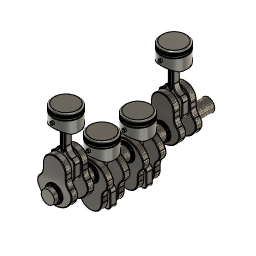
piston v3 (Autodesk Fusion 360 design; units mm, degrees)
Autodesk Fusion 360 part; units mm, degrees
note: some values were not read from the file. Set by a fixed rule: which face or edge a step refers to.
sketch "Sketch1" plane through (0, 0, 0) normal (0, 1, 0) x (1, 0, 0) in component "piston"
  line L0 (0, 0) -> (40, 0)
  line L1 (40, 0) -> (40, -55)
  line L2 (40, -55) -> (0, -55)
  line L3 (0, -55) -> (0, 0)
  line L4 (40, -48) -> (36, -48)
  line L5 (36, -48) -> (36, -46)
  line L6 (36, -46) -> (40, -46)
  line L7 (40, -46) -> (40, -48)
  line L8 (40, -44) -> (36, -44)
  line L9 (36, -44) -> (36, -42)
  line L10 (36, -42) -> (40, -42)
  line L11 (40, -42) -> (40, -44)
  line L12 (40, -38) -> (36, -38)
  line L13 (36, -38) -> (36, -36)
  line L14 (36, -36) -> (40, -36)
  line L15 (40, -36) -> (40, -38)
  dimension "d1" = 55
  dimension "d2" = 40
  dimension "d3" = 7
  dimension "d4" = 2
  dimension "d5" = 4
  dimension "d6" = 2
  dimension "d7" = 2
  dimension "d8" = 2
  dimension "d9" = 4
  dimension "d10" = 4
  dimension "d11" = 4
  constraint horizontal L0
  constraint vertical L1
  constraint horizontal L2
  constraint vertical L3
  constraint coincident L0.start L3.end
  constraint horizontal L4
  constraint vertical L5
  constraint horizontal L6
  constraint vertical L7
  constraint coincident L1 L4.start
  constraint horizontal L8
  constraint vertical L9
  constraint horizontal L10
  constraint vertical L11
  constraint coincident L1 L8.start
  constraint horizontal L12
  constraint vertical L13
  constraint horizontal L14
  constraint vertical L15
  constraint coincident L1 L12.start
  measures "d1" distance of L0.start L2.end
  measures "d2" distance of L0.start L0.end
  measures "d3" distance of L2 L4
  measures "d4" distance of L6 L8
  measures "d5" distance of L10 L12
  measures "d6" distance of L4.end L5.end
  measures "d7" distance of L8.end L9.end
  measures "d8" distance of L12.end L13.end
  measures "d9" distance of L4.start L4.end
  measures "d10" distance of L8.start L8.end
  measures "d11" distance of L12.start L12.end
revolve "Revolve1" add sketch "Sketch1" angle 360 about axis through (0, 0, 55) along (0, 0, -1) contours L0 L1 L2 L3 L4 L5 L6 L8 L9 L10 L12 L13 L14 makes body 1 in component "piston"
fillet "Fillet1" radius 5 1 edges at (-37.2931, -14.4646, 55) on bodies 1 in component "piston"
sketch "Sketch2" plane through (0, 0, 0) normal (0, 0, 1) x (1, 0, 0) in component "piston"
  circle A0 centre (0, 0) radius 35
  dimension "d15" = 70
  constraint coincident A0.centre origin
  measures "d15" diameter of A0
extrude "Extrude1" cut sketch "Sketch2" along normal blind 50 bodies 1 in component "piston"
sketch "Sketch3" plane through (0, 0, 0) normal (0, 1, 0) x (1, 0, 0) in component "piston"
  line L0 (-40, 0) -> (40, 0)
  line L1 (-40, -36) -> (40, -36)
  line L2 (0, 0) -> (0, -10)
  arc A0 (-35.5, 0) -> (35.5, 0) centre (0, 58.0125) ccw
  circle A1 centre (0, -24) radius 5
  dimension "d18" = 4.5
  dimension "d19" = 4.5
  dimension "d20" = 10
  dimension "d21" = 24
  dimension "d22" = 10
  constraint coincident L2.start origin
  constraint perpendicular L0 L2
  constraint coincident L2.end A0
  constraint coincident L0 A0.end
  constraint coincident L0 A0.start
  measures "d18" distance of L0.start A0.start
  measures "d19" distance of L0.end A0.end
  measures "d20" diameter of A1
  measures "d21" distance of L2.start A1.centre
  measures "d22" distance of L2.start L2.end
extrude "Extrude2" cut sketch "Sketch3" along normal mid plane 90 bodies 1 in component "piston"
pattern_linear "R-Pattern1" count 4 spacing 250 along (0, -1, 0) of bodies 1 makes body 2 at (-8.1193, -284.0452, 27.7018) makes body 3 at (-8.1193, -534.0452, 27.7018) makes body 4 at (-8.1193, -784.0452, 27.7018) in component "piston"
sketch "Sketch1 (2)" plane through (0, 0, 0) normal (0, 1, 0) x (1, 0, 0) in component "connecting rod"
  circle A0 centre (0, -50) radius 8.5
  circle A1 centre (0, -50) radius 5
  circle A2 centre (0, 75) radius 22.5
  line L0 (8.5, -50) -> (8.5, 25)
  line L1 (0, 75) -> (36, 75)
  line L2 (36, 75) -> (36, 50)
  line L3 (36, 50) -> (33.5, 50)
  arc A3 (33.5, 50) -> (8.5, 25) centre (33.5, 25) ccw
  line L4 (0, 75) -> (0, 20) construction
  line L5 (-8.5, -50) -> (-8.5, 25)
  arc A4 (-8.5, 25) -> (-33.5, 50) centre (-33.5, 25) ccw
  line L6 (-36, 75) -> (-36, 50)
  line L7 (-36, 50) -> (-33.5, 50)
  line L8 (0, 75) -> (-36, 75)
  line L9 (-36, 75) -> (36, 75)
  line L10 (36, 75) -> (36, 107.5)
  line L11 (36, 107.5) -> (-36, 107.5)
  line L12 (-36, 107.5) -> (-36, 75)
  circle A5 centre (0, -35) radius 4.75
  circle A6 centre (0, 37.5) radius 4.75
  line L13 (-4.75, -35) -> (-4.75, 37.5)
  line L14 (4.75, 37.5) -> (4.75, -35)
  dimension "d29" = 10
  dimension "d30" = 17
  dimension "d31" = 45
  dimension "d32" = 125
  dimension "d33" = 36
  dimension "d34" = 25
  dimension "d35" = 25
  dimension "d36" = 72
  dimension "d37" = 32.5
  dimension "d38" = 9.5
  dimension "d39" = 9.5
  dimension "d40" = 15
  dimension "d41" = 37.5
  constraint concentric A0 A1
  constraint coincident A0 L0.start
  constraint tangent A0 L0
  constraint vertical L0
  constraint coincident A2.centre L1.start
  constraint perpendicular L0 L1
  constraint perpendicular L1 L2
  constraint perpendicular L2 L3
  constraint tangent L3 A3
  constraint tangent L0 A3
  constraint perpendicular L1 L4
  constraint symmetric L0.start L4 L5.start
  constraint symmetric A2.centre L4 L1.start
  constraint symmetric L1.end L4 L6.start
  constraint symmetric L2.end L4 L6.end
  constraint symmetric L3.end L4 A4.end
  constraint symmetric L0.end L4 L5.end
  constraint symmetric A3 L4 A4
  constraint horizontal L9
  constraint vertical L10
  constraint horizontal L11
  constraint vertical L12
  constraint coincident A5 L13.start
  constraint coincident A6 L13.end
  constraint tangent A6 L13
  constraint parallel L5 L13
  constraint coincident A6 L14.start
  constraint coincident A5 L14.end
  constraint tangent A5 L14
  constraint parallel L0 L14
  measures "d29" diameter of A1
  measures "d30" diameter of A0
  measures "d31" diameter of A2
  measures "d32" distance of A0.centre A2.centre
  measures "d33" distance of A2.centre L1.end
  measures "d34" distance of L1.end L2.end
  measures "d35" radius of A3
  measures "d36" distance of L6.start L1.end
  measures "d37" distance of L6.start L11.end
  measures "d38" diameter of A5
  measures "d39" diameter of A6
  measures "d40" distance of A0.centre A5.centre
  measures "d41" distance of A2.centre A6.centre
extrude "Extrude1'" add sketch "Sketch1 (2)" along normal mid plane 20 separate body contours A0 | A0 A2 L0 L1 L2 L3 A3 L5 A4 L6 L7 L8 L9 | A2 L1 L8 L9 L10 L11 L12 makes body 5 in component "connecting rod"
extrude "Extrude2'" add sketch "Sketch1 (2)" along normal mid plane 10 contours A5 | A5 A6 L13 L14 | A6 bodies 5 in component "connecting rod"
fillet "Fillet1'" radius 12.5 4 edges at (36, 0, -50) (36, 0, -107.5) (-36, 0, -107.5) (-36, 0, -50) on bodies 5 in component "connecting rod"
fillet "Fillet2" chord length 2.5 24 edges at (0, -10, 58.5) (-8.5, -10, 12.5) (-13.6044, -10, -40.1383) (-33.4478, -10, -53.573) (-36, -10, -78.071) (-32.3388, -10, -103.8388) (0, -10, -107.5) (32.3388, -10, -103.8388) (36, -10, -78.071) (33.4478, -10, -53.573) (13.6044, -10, -40.1383) (8.5, -10, 12.5) (33.4478, 10, -53.573) (36, 10, -78.071) (32.3388, 10, -103.8388) (0, 10, -107.5) (-32.3388, 10, -103.8388) (-36, 10, -78.071) (-33.4478, 10, -53.573) (-13.6044, 10, -40.1383) (-8.5, 10, 12.5) (0, 10, 58.5) (8.5, 10, 12.5) (13.6044, 10, -40.1383) on bodies 5 in component "connecting rod"
fillet "Fillet3" chord length 1.5 16 edges at (4.75, -5, -1.25) (0, -5, -42.25) (-4.75, -5, -1.25) (0, -5, 39.75) (4.75, -10, -1.25) (0, -10, -42.25) (-4.75, -10, -1.25) (0, -10, 39.75) (4.75, 5, -1.25) (0, 5, 39.75) (-4.75, 5, -1.25) (0, 5, -42.25) (4.75, 10, -1.25) (0, 10, 39.75) (-4.75, 10, -1.25) (0, 10, -42.25) on bodies 5 in component "connecting rod"
sketch "Sketch1 (3)" plane through (0, 0, 0) normal (0, 1, 0) x (1, 0, 0) in component "pin"
cylinder "CylinderPrimitive1" add diameter 10 height 90 placed x (1, 0, 0) y (0, 0, -1) z (0, 1, 0) at (75, 0, 175) separate body makes body 6 in component "pin"
fillet "Fillet1''" radius 1.5 2 edges at (70.3384, 90, 176.8081) (70.3384, 0, 173.1919) on bodies 6 in component "pin"
pattern_linear "R-Pattern1'" count 4 spacing 200 along (0, -1, 0) of bodies 6 makes body 7 at (70.3015, -169.5, 176.7101) makes body 8 at (70.3015, -369.5, 176.7101) makes body 9 at (70.3015, -569.5, 176.7101) in component "pin"
sketch "Sketch1 (4)" plane through (0, 0, 0) normal (0, 1, 0) x (1, 0, 0) in component "crank shaft"
  circle A0 centre (0, 75) radius 22.5
  circle A1 centre (0, 75) radius 35
  circle A2 centre (0, 10.5) radius 20
  circle A3 centre (0, 10.5) radius 25
  arc A4 (-55, 32.5) -> (55, 32.5) centre (0, 32.5) ccw
  line L0 (35, 75) -> (35, 32.5)
  line L1 (-35, 75) -> (-35, 32.5)
  line L2 (-35, 32.5) -> (-55, 32.5)
  line L3 (35, 32.5) -> (55, 32.5)
  dimension "d64" = 70
  dimension "d65" = 110
  dimension "d66" = 40
  dimension "d67" = 50
  dimension "d68" = 42.5
  dimension "d69" = 22
  constraint concentric A0 A1
  constraint concentric A2 A3
  constraint coincident A1 L0.start
  constraint tangent A1 L0
  constraint coincident A1 L1.start
  constraint tangent A1 L1
  measures "d64" diameter of A1
  measures "d65" diameter of A4
  measures "d66" diameter of A2
  measures "d67" diameter of A3
  measures "d68" distance of A0.centre A4.centre
  measures "d69" distance of A4.centre A2.centre
extrude "Extrude1''" add sketch "Sketch1 (4)" against normal blind 20 from surface at -15 separate body contours A0 | A1 | A1 A4 L0 L1 L2 L3 | A2 | A3 makes body 10 in component "crank shaft"
extrude "Extrude2''" add sketch "Sketch1 (4)" against normal blind 20 from surface at -35 contours A2 bodies 10 in component "crank shaft"
extrude "Extrude3" add sketch "Sketch1 (4)" against normal blind 5 from surface at -35 contours A3 bodies 10 in component "crank shaft"
fillet "Fillet1'''" radius 30 2 edges at (35, -25, -32.5) (-35, -25, -32.5) on bodies 10 in component "crank shaft"
fillet "Fillet2'" radius 25 2 edges at (55, -25, -32.5) (-55, -25, -32.5) on bodies 10 in component "crank shaft"
fillet "Fillet3'" chord length 2.5 16 edges at (-51.987, -35, -25.6375) (-37.4915, -35, -48.8142) (-35, -35, -67.8921) (0, -35, -110) (35, -35, -67.8921) (37.4915, -35, -48.8142) (51.987, -35, -25.6375) (0, -35, 22.5) (51.987, -15, -25.6375) (37.4915, -15, -48.8142) (35, -15, -67.8921) (0, -15, -110) (-35, -15, -67.8921) (-37.4915, -15, -48.8142) (-51.987, -15, -25.6375) (0, -15, 22.5) on bodies 10 in component "crank shaft"
fillet "Fillet4" chord length 1.5 3 edges at (-18.6465, -40, -17.7323) (-23.3082, -40, -19.5404) (-23.3082, -35, -1.4596) on bodies 10 in component "crank shaft"
mirror "Mirror1" about plane through (0, 0, 0) normal (0, 1, 0) of bodies 10 makes body 11 in component "crank shaft"
extrude "Extrude4" add sketch "Sketch1 (4)" along normal blind 15 contours A0 bodies 11 in component "crank shaft"
extrude "Extrude5" add sketch "Sketch1 (4)" against normal blind 15 contours A0 bodies 10 11 in component "crank shaft"
pattern_linear "R-Pattern1''" count 4 spacing 110 along (0, 1, 0) of bodies 10 makes body 12 at (26.9012, 95, -28.8147) makes body 13 at (26.9012, 205, -28.8147) makes body 14 at (26.9012, 315, -28.8147) in component "crank shaft"
move_body "Move1" bodies 12 13 to x (-1, 0, 0) y (0, 1, 0) z (0, 0, -1) at (0, 0, -21) in component "crank shaft"
combine "Combine1" operation add target body 10 tool bodies 12 13 14 in component "crank shaft"
extrude "Extrude6" add 1 faces at (4.8168, 385, -2.3952) along direction (0, 1, 0) blind 50 on bodies 10 bodies 10 in component "crank shaft"
sketch "Sketch1 (5)" plane through (0, 435, 0) normal (0, 1, 0) x (-1, 0, 0)
  circle A0 centre (0, -10.5) radius 20
  circle A1 centre (0, -10.5) radius 37.5
  dimension "d99" = 75
  constraint concentric A0 A1
  measures "d99" diameter of A1
extrude "Extrude1'''" add sketch "Sketch1 (5)" against normal blind 20 separate body makes body 15 in component "Component"
copy_body "CopyPasteBodies1" bodies 5 body 5 seen with x (1, 0, 0) y (0, 1, 0) z (0, 0, 1) at (-45.7777, -70.7188, -15.1444) makes body 16 in component "connecting rod2"
move_body "Move1'" bodies 16 to x (1, 0, 0) y (0, 1, 0) z (0, 0, 1) at (-58.0098, 0, -39.7474) in component "connecting rod2"
copy_body "CopyPasteBodies1'" bodies 5 body 5 seen with x (1, 0, 0) y (0, 1, 0) z (0, 0, 1) at (-101.0736, -178.6533, -36.6467) makes body 17 in component "Component'"
move_body "Move1''" bodies 17 to x (1, 0, 0) y (0, 1, 0) z (0, 0, 1) at (0, -102.1146, 13.7993) in component "Component'"
copy_body "CopyPasteBodies1''" bodies 5 body 5 seen with x (1, 0, 0) y (0, 1, 0) z (0, 0, 1) at (-101.0736, -178.6533, -36.6467) makes body 18 in component "Component''"
move_body "Move1'''" bodies 18 to x (1, 0, 0) y (0, 1, 0) z (0, 0, 1) at (0, -250.0427, 33.6702) in component "Component''"
copy_body "CutPasteBodies1" bodies 2 body 2 seen with x (1, 0, 0) y (0, 1, 0) z (0, 0, 1) at (-155.4399, -103.1423, 107.5542) removing the originals makes body 19 in component "Component'''"
copy_body "CutPasteBodies1'" bodies 3 body 3 seen with x (1, 0, 0) y (0, 1, 0) z (0, 0, 1) at (-155.4399, -103.1423, 107.5542) removing the originals makes body 20 in component "Component''''"
copy_body "CutPasteBodies1''" bodies 4 body 4 seen with x (1, 0, 0) y (0, 1, 0) z (0, 0, 1) at (-155.4399, -103.1423, 107.5542) removing the originals makes body 21 in component "Component'''''"
copy_body "CutPasteBodies1'''" bodies 7 body 7 seen with x (1, 0, 0) y (0, 1, 0) z (0, 0, 1) at (-134.4515, -29.966, 131.6173) removing the originals makes body 22 in component "Component''''''"
copy_body "CutPasteBodies1''''" bodies 8 body 8 seen with x (1, 0, 0) y (0, 1, 0) z (0, 0, 1) at (-134.4515, -29.966, 131.6173) removing the originals makes body 23 in component "Component'''''''"
copy_body "CutPasteBodies1'''''" bodies 9 body 9 seen with x (1, 0, 0) y (0, 1, 0) z (0, 0, 1) at (-134.4515, -29.966, 131.6173) removing the originals makes body 24 in component "Component''''''''"
sketch "Sketch2 (2)" plane through (0, 0, 210) normal (0, 0, 1) x (-1, 0, 0)
  circle A0 centre (0, -142.4749) radius 35
  line L0 (170.6537, -489.8535) -> (-175, -489.8535)
  line L1 (-175, -489.8535) -> (-175, 75)
  line L2 (-175, 75) -> (170.6537, 75)
  line L3 (170.6537, 75) -> (170.6537, -489.8535)
  circle A1 centre (0, -32.4749) radius 40
  circle A2 centre (0, -142.4749) radius 40
  circle A3 centre (0, -252.4749) radius 40
  circle A4 centre (0, -362.4749) radius 40
  constraint horizontal L0
  constraint vertical L1
  constraint horizontal L2
  constraint vertical L3
extrude "Extrude1''''" add sketch "Sketch2 (2)" along normal blind 25 separate body contours L0 L1 L2 L3 makes body 25 in component "Component'''''''''"
component "pistons" placed x (1, 0, 0) y (0, 1, 0) z (0, 0, 1) at (0, 0, 0)
component "connecting rods" placed x (1, 0, 0) y (0, 1, 0) z (0, 0, 1) at (0, 0, 0)
component "pins" placed x (1, 0, 0) y (0, 1, 0) z (0, 0, 1) at (0, 0, 0)
component "crank shaft" placed x (-1, 0, 0) y (0, 1, 0) z (0, 0, -1) at (0, 31.9725, -21)
component "Component" placed x (1, 0, 0) y (0, 1, 0) z (0, 0, 1) at (0, 0, 0)
component "Component'''''''''" placed x (1, 0, 0) y (0, 1, 0) z (0, 0, 1) at (0, 0, 0)
component "piston" placed x (1, 0, 0) y (0, 1, 0) z (0, 0, 1) at (0, 252.4749, 26) in component "pistons"
component "Component'''" placed x (1, 0, 0) y (0, 1, 0) z (0, 0, 1) at (155.4399, 715.6171, 47.4458) in component "pistons"
component "Component''''" placed x (1, 0, 0) y (0, 1, 0) z (0, 0, 1) at (155.4399, 745.6171, -81.5542) in component "pistons"
component "Component'''''" placed x (1, 0, 0) y (0, 1, 0) z (0, 0, 1) at (155.4399, 885.6171, 47.4458) in component "pistons"
component "connecting rod" placed x (1, 0, 0) y (0, 1, 0) z (0, 0, 1) at (0, 141.9725, 0) in component "connecting rods"
component "connecting rod2" placed x (1, 0, 0) y (0, 1, 0) z (0, 0, 1) at (103.7875, 102.6913, 183.8918) in component "connecting rods"
component "Component'" placed x (1, 0, 0) y (0, 1, 0) z (0, 0, 1) at (101.0736, 532.7404, 22.8474) in component "connecting rods"
component "Component''" placed x (1, 0, 0) y (0, 1, 0) z (0, 0, 1) at (101.0736, 790.6685, 131.9765) in component "connecting rods"
component "pin" placed x (1, 0, 0) y (0, 1, 0) z (0, 0, 1) at (-75, 96.9725, -125) in component "pins"
component "Component''''''" placed x (1, 0, 0) y (0, 1, 0) z (0, 0, 1) at (59.4515, 216.9385, -127.6173) in component "pins"
component "Component'''''''" placed x (1, 0, 0) y (0, 1, 0) z (0, 0, 1) at (59.4515, 636.9385, -256.6173) in component "pins"
component "Component''''''''" placed x (1, 0, 0) y (0, 1, 0) z (0, 0, 1) at (59.4515, 946.9385, -127.6173) in component "pins"
equation "d7 = d6"
equation "d8 = d6"
equation "d10 = d9"
equation "d11 = d9"
